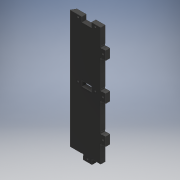
# Autodesk Inventor part: BA03
Saved by Autodesk Inventor 2017 (Build 210142000, 142)
## iProperties
Created: 2019-05-22
Part Number: BA03
Material: Wood (Cherry)
Document SubType Name: Modeling
Designer: Dell
Density: 0.63 g/cm^3
Appearance: Smooth - Black
Mass: 240.222 g
Surface Area: 757.429 cm^2
Volume: 381.304 cm^3
Author: Dell
Autodesk Inventor part; units mm, degrees
ref_plane "YZ Plane" through (0, 0, 0) normal (1, 0, 0) x (0, 1, 0)
ref_plane "XZ Plane" through (0, 0, 0) normal (0, 1, 0) x (-1, 0, 0)
ref_plane "XY Plane" through (0, 0, 0) normal (0, 0, 1) x (1, 0, 0)
sketch "Sketch1" plane through (0, 0, 0) normal (0, 0, 1) x (1, 0, 0)
  line L0 (0, 0) -> (88.9, 0)
  line L1 (88.9, 0) -> (88.9, 12.7)
  line L2 (88.9, 12.7) -> (7.3323, 12.7)
  line L3 (7.3323, 12.7) -> (0, 0)
  dimension "d0" = 88.9
  dimension "d1" = 12.7
  dimension "d2" = 60
  constraints: 8 end point, 2 perpendicular, 1 horizontal
  measures "d0" distance of L0.start L0.end
  measures "d1" distance of L0.end L1.end
  measures "d2" angle of L0 L3
extrude "Extrusion1" add sketch "Sketch1" along normal blind 342.9
sketch "Sketch2" plane through (0, 0, 0) normal (0, -1, 0) x (1, 0, 0)
  line L0 (38.1, 342.9) -> (63.5, 342.9)
  line L1 (63.5, 342.9) -> (63.5, 355.6)
  line L2 (63.5, 355.6) -> (38.1, 355.6)
  line L3 (38.1, 355.6) -> (38.1, 342.9)
  line L4 (0, 342.9) -> (101.6, 342.9)
  line L5 (0, 342.9) -> (88.9, 342.9) projected
  point P0 (0, 0)
  point P1 (50.8, 342.9)
  dimension "d5" = 25.4
  dimension "d6" = 12.7
  dimension "d9" = 101.6
  constraints: 10 end point, 2 midpoint, 2 parallel, 1 collinear, 1 horizontal, 1 perpendicular
  measures "d5" distance of L2.end L1.end
  measures "d6" distance of L1.end L0.end
  measures "d9" distance of L4.start L4.end
extrude "Extrusion2" add sketch "Sketch2" against normal blind 12.7
sketch "Sketch3" plane through (0, 0, 0) normal (0, -1, 0) x (1, 0, 0)
  line L0 (63.5, 342.9) -> (63.5, 355.6) projected
  line L1 (63.5, 355.6) -> (38.1, 355.6) projected
  circle A0 centre (50.8, 349.25) radius 2.25
  point P0 (0, 0)
  point P1 (50.8, 355.6)
  point P2 (63.5, 349.25)
  dimension "d10" = 4.5
  constraints: 2 midpoint, 1 centre point, 1 horizontal alignment, 1 vertical alignment
  measures "d10" diameter of A0
extrude "Extrusion3" cut sketch "Sketch3" against normal through all
sketch "Sketch4" plane through (0, 0, 0) normal (0, -1, 0) x (1, 0, 0)
  line L0 (88.9, 0) -> (88.9, 342.9) projected
  line L1 (88.9, 50.8) -> (101.6, 50.8)
  line L2 (101.6, 50.8) -> (101.6, 76.2)
  line L3 (101.6, 76.2) -> (88.9, 76.2)
  line L4 (88.9, 76.2) -> (88.9, 50.8)
  line L5 (88.9, 292.1) -> (101.6, 292.1)
  line L6 (101.6, 292.1) -> (101.6, 266.7)
  line L7 (101.6, 266.7) -> (88.9, 266.7)
  line L8 (88.9, 266.7) -> (88.9, 292.1)
  line L9 (88.9, 184.15) -> (101.6, 184.15)
  line L10 (101.6, 184.15) -> (101.6, 158.75)
  line L11 (101.6, 158.75) -> (88.9, 158.75)
  line L12 (88.9, 158.75) -> (88.9, 184.15)
  circle A0 centre (95.25, 279.4) radius 2.25
  circle A1 centre (95.25, 171.45) radius 2.25
  circle A2 centre (95.25, 63.5) radius 2.25
  point P0 (0, 0)
  point P1 (88.9, 171.45)
  point P2 (95.25, 292.1)
  point P3 (95.25, 184.15)
  point P4 (95.25, 76.2)
  point P5 (101.6, 279.4)
  point P6 (101.6, 171.45)
  point P7 (101.6, 63.5)
  dimension "d13" = 12.7
  dimension "d14" = 25.4
  dimension "d15" = 12.7
  dimension "d16" = 25.4
  dimension "d17" = 12.7
  dimension "d18" = 25.4
  dimension "d19" = 50.8
  dimension "d20" = 50.8
  dimension "d21" = 4.5
  dimension "d22" = 4.5
  dimension "d23" = 4.5
  constraints: 24 end point, 8 midpoint, 6 parallel, 3 centre point, 3 horizontal, 3 horizontal alignment, 3 perpendicular, 3 point on line, 3 vertical alignment
  measures "d13" distance of L3.end L2.end
  measures "d14" distance of L2.end L1.end
  measures "d15" distance of L6.end L7.end
  measures "d16" distance of L5.end L6.end
  measures "d17" distance of L10.end L11.end
  measures "d18" distance of L9.end L10.end
  measures "d19" distance from line of L0.end L5
  measures "d20" distance from line of L0.start L1
  measures "d21" diameter of A0
  measures "d22" diameter of A1
  measures "d23" diameter of A2
extrude "Extrusion4" add sketch "Sketch4" against normal blind 12.7
sketch "Sketch9" plane through (88.9, 0, 292.1) normal (0, 0, 1) x (1, 0, 0)
  line L0 (-88.9, 0) -> (0, 0) projected
  line L1 (-88.9, 0) -> (-88.9, 12.7)
  line L2 (0, 12.7) -> (-81.5677, 12.7) projected
  line L3 (-88.9, 12.7) -> (-81.5677, 12.7)
  line L4 (-81.5677, 12.7) -> (-88.9, 0)
  line L5 (-81.5677, 12.7) -> (-88.9, 0) projected
  constraints: 6 end point, 1 horizontal, 1 vertical
extrude "Extrusion9" [suppressed]
sketch "Sketch10" plane through (88.9, 0, 184.15) normal (0, 0, 1) x (1, 0, 0)
  line L0 (-81.5677, 12.7) -> (-88.9, 0) projected
  line L1 (-81.5677, 12.7) -> (-88.9, 12.7) projected
  line L2 (-88.9, 12.7) -> (-88.9, 0) projected
  point P0 (-88.9, 0)
extrude "Extrusion10" [suppressed]
sketch "Sketch11" plane through (88.9, 0, 76.2) normal (0, 0, 1) x (1, 0, 0)
  line L0 (-81.5677, 12.7) -> (-88.9, 0) projected
  line L1 (-81.5677, 12.7) -> (-88.9, 12.7) projected
  line L2 (-88.9, 12.7) -> (-88.9, 0) projected
extrude "Extrusion11" [suppressed]
ref_plane "Work Plane1" through (0, 0, 171.45) normal (0, 0, 1) x (1, 0, 0)
mirror "Mirror1" about plane through (0, 0, 171.45) normal (0, 0, 1) of "Extrusion1", "Extrusion2", "Extrusion3", "Extrusion4"
sketch "Sketch12" plane through (7.3323, 12.7, 342.9) normal (0, 1, 0) x (1, 0, 0)
  line L0 (56.1677, 0) -> (56.1677, -12.7) projected
  line L1 (56.1677, -12.7) -> (56.1677, 0) projected
  line L2 (56.1677, -12.7) -> (30.7677, -12.7) projected
  line L3 (30.7677, -12.7) -> (56.1677, -12.7) projected
  line L4 (30.7677, 0) -> (30.7677, -12.7) projected
  line L5 (56.1677, 0) -> (30.7677, 0)
  line L6 (81.5677, 0) -> (56.1677, 0) projected
  line L7 (30.7677, -12.7) -> (56.1677, -12.7)
  line L8 (56.1677, -12.7) -> (56.1677, 0)
  line L9 (56.1677, 0) -> (30.7677, 0)
  line L10 (30.7677, 0) -> (30.7677, -12.7)
  point P0 (-7.3323, 342.9)
  constraints: 10 end point, 2 horizontal, 2 parallel, 1 perpendicular
extrude "Extrusion12" cut sketch "Sketch12" along normal through all both and the other way through all
sketch "Sketch13" plane through (7.3323, 12.7, 342.9) normal (0, 1, 0) x (1, 0, 0)
  circle A0 centre (15.7838, 6.35) radius 2.25
  line L0 (81.5677, 0) -> (0, 0) projected
  circle A1 centre (65.7838, 6.35) radius 2.25
  line L1 (28.0838, 0) -> (53.4838, 0)
  line L2 (53.4838, 0) -> (53.4838, 12.7)
  line L3 (53.4838, 12.7) -> (28.0838, 12.7)
  line L4 (28.0838, 12.7) -> (28.0838, 0)
  line L5 (15.7838, 6.35) -> (65.7838, 6.35) construction
  point P0 (-7.3323, 342.9)
  point P1 (40.7838, 6.35)
  point P2 (40.7838, 0)
  point P3 (40.7838, 0)
  dimension "d44" = 4.5
  dimension "d45" = 6.35
  dimension "d46" = 4.5
  dimension "d47" = 25.4
  dimension "d48" = 12.7
  dimension "d49" = 50
  constraints: 10 end point, 5 midpoint, 2 centre point, 2 horizontal, 2 parallel, 1 perpendicular, 1 vertical alignment
  measures "d44" diameter of A0
  measures "d45" distance from line of L0 L5.start
  measures "d46" diameter of A1
  measures "d47" distance of L3.end L2.end
  measures "d48" distance of L2.end L1.end
  measures "d49" distance of L5.start L5.end
extrude "Extrusion13" cut sketch "Sketch13" against normal through all
sketch "Sketch14" plane through (88.9, 0, 50.8) normal (0, -1, 0) x (1, 0, 0)
  line L0 (12.7, 107.95) -> (12.7, 133.35) projected
  line L1 (-28.0838, 279.4) -> (-53.4838, 279.4) projected
  line L2 (-53.4838, 130.65) -> (-28.0838, 130.65)
  line L3 (-28.0838, 130.65) -> (-28.0838, 117.95)
  line L4 (-28.0838, 117.95) -> (-53.4838, 117.95)
  line L5 (-53.4838, 117.95) -> (-53.4838, 130.65)
  point P0 (-88.9, -50.8)
  dimension "d54" = 12.7
  dimension "d55" = 10
  constraints: 8 end point, 2 parallel, 2 vertical alignment, 1 horizontal, 1 perpendicular
  measures "d54" distance of L4.end L2.start
  measures "d55" distance from line of L0.start L4
extrude "Extrusion14" cut sketch "Sketch14" against normal through all
sketch "Sketch15" plane through (88.9, 0, 50.8) normal (0, -1, 0) x (1, 0, 0)
  circle A0 centre (-65.7838, 124.3) radius 2.25
  circle A1 centre (-15.7838, 124.3) radius 2.25
  circle A2 centre (-65.7838, 285.75) radius 2.25 projected
  circle A3 centre (-15.7838, 285.75) radius 2.25 projected
  line L0 (-28.0838, 130.65) -> (-28.0838, 117.95) projected
  point P0 (-88.9, -50.8)
  point P1 (-28.0838, 124.3)
  point P2 (-28.0838, 124.3)
  dimension "d56" = 4.5
  dimension "d57" = 4.5
  constraints: 2 centre point, 2 horizontal alignment, 2 midpoint, 2 vertical alignment
  measures "d56" diameter of A0
  measures "d57" diameter of A1
extrude "Extrusion15" cut sketch "Sketch15" against normal through all contours A0 | A1
sketch "Sketch16" plane through (88.9, 12.7, 292.1) normal (0, 1, 0) x (1, 0, 0)
  line L0 (-54.7538, 124.62) -> (-26.8138, 124.62)
  line L1 (-26.8138, 124.62) -> (-26.8138, 109.38)
  line L2 (-26.8138, 109.38) -> (-54.7538, 109.38)
  line L3 (-54.7538, 109.38) -> (-54.7538, 124.62)
  line L4 (-88.9, -50.8) -> (-53.4838, -50.8) projected
  line L5 (-54.7538, -50.8) -> (-26.8138, -50.8)
  line L6 (-26.8138, -50.8) -> (-26.8138, -36.83)
  line L7 (-26.8138, -36.83) -> (-54.7538, -36.83)
  line L8 (-54.7538, -36.83) -> (-54.7538, -50.8)
  line L9 (-28.0838, 110.65) -> (-53.4838, 110.65) projected
  line L10 (-53.4838, -38.1) -> (-28.0838, -38.1) projected
  line L11 (-53.4838, 110.65) -> (-53.4838, 123.35) projected
  circle A0 centre (-53.0451, 294.3451) radius 3.175
  circle A1 centre (-23.1549, 294.3451) radius 3.175
  circle A2 centre (2.2451, 243.5451) radius 3.175
  circle A3 centre (2.2451, 213.6549) radius 3.175
  circle A4 centre (2.2451, 135.5951) radius 3.175
  circle A5 centre (2.2451, 105.7049) radius 3.175
  circle A6 centre (2.2451, 27.6451) radius 3.175
  circle A7 centre (2.2451, -2.2451) radius 3.175
  line L12 (-53.0451, 294.3451) -> (-50.8, 292.1)
  line L13 (-50.8, 304.8) -> (-50.8, 292.1) projected
  line L14 (0, 241.3) -> (2.2451, 243.5451)
  line L15 (12.7, 241.3) -> (0, 241.3) projected
  point P0 (-88.9, 292.1)
  point P1 (-40.7838, 110.65)
  point P2 (-40.7838, 109.38)
  point P3 (-40.7838, -36.83)
  point P4 (-40.7838, -38.1)
  point P5 (-53.4838, 117)
  point P6 (-54.7538, 117)
  point P7 (0, 0)
  point P8 (0, 25.4)
  point P9 (0, 107.95)
  point P10 (0, 133.35)
  point P11 (0, 215.9)
  point P12 (-25.4, 292.1)
  dimension "d63" = 6.35
  dimension "d64" = 6.35
  dimension "d65" = 6.35
  dimension "d66" = 6.35
  dimension "d67" = 6.35
  dimension "d68" = 6.35
  dimension "d69" = 6.35
  dimension "d70" = 6.35
  dimension "d60" = 1.27
  dimension "d61" = 1.27
  dimension "d62" = 1.27
  dimension "d77" = 45
  dimension "d78" = 45
  constraints: 20 end point, 9 vertical alignment, 6 midpoint, 4 parallel, 3 coincident, 3 point on line, 2 horizontal, 2 horizontal alignment, 2 perpendicular, 24 other
  measures "d60" distance between parallel lines of L2 L9
  measures "d61" distance between parallel lines of L3 L11
  measures "d62" distance between parallel lines of L7 L10
  measures "d77" angle of L13 L12
  measures "d78" angle of L14 L15
extrude "Extrusion16" cut sketch "Sketch16" against normal through all
sketch "Sketch17" plane through (101.6, 12.7, 292.1) normal (0, 1, 0) x (1, 0, 0)
  line L0 (-63.5, 304.8) -> (-38.1, 304.8)
  line L1 (-38.1, 304.8) -> (-38.1, 306.07)
  line L2 (-38.1, 306.07) -> (-63.5, 306.07)
  line L3 (-63.5, 306.07) -> (-63.5, 304.8)
  line L4 (0, 241.3) -> (1.27, 241.3)
  line L5 (1.27, 241.3) -> (1.27, 215.9)
  line L6 (1.27, 215.9) -> (0, 215.9)
  line L7 (0, 215.9) -> (0, 241.3)
  line L8 (0, 133.35) -> (1.27, 133.35)
  line L9 (1.27, 133.35) -> (1.27, 107.95)
  line L10 (1.27, 107.95) -> (0, 107.95)
  line L11 (0, 107.95) -> (0, 133.35)
  line L12 (0, 25.4) -> (1.27, 25.4)
  line L13 (1.27, 25.4) -> (1.27, 0)
  line L14 (1.27, 0) -> (0, 0)
  line L15 (0, 0) -> (0, 25.4)
  point P0 (-101.6, 292.1)
  dimension "d73" = 1.27
  dimension "d74" = 1.27
  constraints: 32 end point, 8 parallel, 4 coincident, 4 horizontal, 4 perpendicular, 1 point on line, 1 vertical alignment
  measures "d73" distance between parallel lines of L2 L0
  measures "d74" distance of L4.start L4.end
extrude "Extrusion17" add sketch "Sketch17" against normal up to surface (12.7 mm away) from surface at 0
equation "\"d1\" = Panel_Thickness"
equation "\"d6\" = Panel_Thickness"
equation "\"d13\" = Panel_Thickness"
equation "\"d15\" = Panel_Thickness"
equation "\"d17\" = Panel_Thickness"
equation "\"d48\" = Panel_Thickness"
equation "\"d54\" = Panel_Thickness"
equation "\"d63\" = Tool_Dia"
equation "\"d64\" = d63"
equation "\"d65\" = d63"
equation "\"d66\" = d63"
equation "\"d67\" = d63"
equation "\"d68\" = d63"
equation "\"d69\" = d63"
equation "\"d70\" = d63"
equation "\"d60\" = Fit_Tolerance"
equation "\"d61\" = Fit_Tolerance"
equation "\"d62\" = Fit_Tolerance"
equation "\"d73\" = Fit_Tolerance"
equation "\"d74\" = d73"
equation "\"Panel_Thickness\" = 12.7"
equation "\"Fit_Tolerance\" = 1.27"
equation "\"Tool_Dia\" = 6.35"
body "Solid1"
